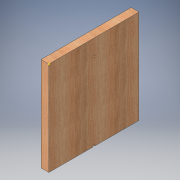
# Autodesk Inventor part: ThickLegOutlet
Saved by Autodesk Inventor 2016 (Build 200138000, 138)
## iProperties
Created: 2016-02-14
Part Number: ThickLegOutlet
Material: Wood (Birch)
Document SubType Name: Modeling
Designer: ron
Density: 0.55 g/cm^3
Appearance: Birch - Natural Polished
Author: ron
Autodesk Inventor part; units mm, degrees
ref_plane "YZ Plane" through (0, 0, 0) normal (1, 0, 0) x (0, 1, 0)
ref_plane "XZ Plane" through (0, 0, 0) normal (0, 1, 0) x (-1, 0, 0)
ref_plane "XY Plane" through (0, 0, 0) normal (0, 0, 1) x (1, 0, 0)
sketch "Sketch1" plane through (0, 0, 0) normal (0, 1, 0) x (-1, 0, 0)
  line L0 (0, 0) -> (50.8, 0)
  line L1 (50.8, 0) -> (50.8, -584.6064)
  line L2 (50.8, -584.6064) -> (0, -584.6064)
  line L3 (0, -584.6064) -> (0, 0)
  dimension "d0" = 584.6064
  dimension "d1" = 50.8
  constraints: 8 end point, 2 parallel, 1 horizontal, 1 perpendicular
  measures "d0" distance of L0.end L1.end
  measures "d1" distance of L1.end L2.end
extrude "Extrusion1" add sketch "Sketch1" along normal blind 609.6
sketch "Sketch2" plane through (0, 609.6, 0) normal (0, 1, 0) x (1, 0, 0)
  point P0 (0, 0)
sketch "Sketch3" plane through (0, 0, 0) normal (1, 0, 0) x (0, 0, -1)
  line L0 (0, 609.6) -> (0, 505.3076)
  line L1 (0, 0) -> (0, 609.6) projected
  line L2 (0, 505.3076) -> (292.3032, 505.3076)
  dimension "d4" = 104.2924
  dimension "d5" = 292.3032
  constraints: 4 end point, 1 horizontal, 1 point on line
  measures "d4" distance of L0.start L0.end
  measures "d5" distance of L0.end L2.end
hole "Hole1" at (0, 505.3076, -292.3032) direction (-1, 0, 0) diameter 12.7 depth 31.75 tip angle 118
sketch "Sketch4" plane through (0, 0, 0) normal (1, 0, 0) x (0, 0, -1)
  line L0 (0, 0) -> (292.3032, 0)
  line L1 (584.6064, 0) -> (0, 0) projected
  line L2 (292.3032, 0) -> (292.3032, 3.175)
  dimension "d13" = 292.3032
  dimension "d14" = 3.175
  constraints: 4 end point, 1 midpoint, 1 vertical
  measures "d13" distance of L0.start L0.end
  measures "d14" distance of L0.end L2.end
hole "Hole2" at (0, 3.175, -292.3032) direction (-1, 0, 0) diameter 12.7 depth 31.75 tip angle 118
sketch "Sketch5" plane through (0, 0, 0) normal (0, -1, 0) x (1, 0, 0)
  line L0 (0, 0) -> (-25.4, 0)
  line L1 (0, 0) -> (-50.8, 0) projected
  line L2 (-25.4, -292.3032) -> (-25.4, 0)
  dimension "d22" = 292.3032
  constraints: 4 end point, 1 midpoint, 1 perpendicular
  measures "d22" distance of L2.start L0.end
hole "Hole3" at (-25.4, 0, -292.3032) direction (0, 1, 0) diameter 12.7 end up to face face through (-15.875, 505.3076, -292.3032) facing (1, 0, 0) round with radius 6.35 far side yes
body "Solid1"
